Autodesk Fusion 360 part; units mm, degrees
(part 40 of 40)
  line L11757 (236.7591, 85.2532) -> (236.7374, 85.0889) construction
  line L11758 (236.7374, 85.0889) -> (236.7148, 84.9245) construction
  line L11759 (236.7148, 84.9245) -> (236.6913, 84.76) construction
  line L11760 (236.6913, 84.76) -> (236.667, 84.5954) construction
  line L11761 (236.667, 84.5954) -> (236.6418, 84.4308) construction
  line L11762 (236.6418, 84.4308) -> (236.6159, 84.266) construction
  line L11763 (236.6159, 84.266) -> (236.5891, 84.1013) construction
  line L11764 (236.5891, 84.1013) -> (236.5614, 83.9364) construction
  line L11765 (236.5614, 83.9364) -> (236.533, 83.7715) construction
  line L11766 (236.533, 83.7715) -> (236.5038, 83.6065) construction
  line L11767 (236.5038, 83.6065) -> (236.4737, 83.4415) construction
  line L11768 (236.4737, 83.4415) -> (236.4428, 83.2764) construction
  line L11769 (236.4428, 83.2764) -> (236.4112, 83.1113) construction
  line L11770 (236.4112, 83.1113) -> (236.3852, 82.9792) construction
  line L11771 (236.3852, 82.9792) -> (236.3654, 82.8801) construction
  line L11772 (236.3654, 82.8801) -> (236.352, 82.814) construction
  line L11773 (236.352, 82.814) -> (236.3452, 82.7809) construction
  arc A310 (232.0535, 81.3864) -> (236.3452, 82.7809) centre (212.132, 150) ccw
  arc A311 (170.3188, 110.6216) -> (172.7536, 108.1868) centre (212.132, 150) ccw
  arc A312 (144.9129, 174.2132) -> (143.5184, 169.9215) centre (212.132, 150) ccw
  arc A313 (253.9452, 189.3784) -> (251.5104, 191.8132) centre (212.132, 150) ccw
  arc A314 (204.8514, 206.9737) -> (201.4504, 206.435) centre (212.132, 150) ccw
  arc A315 (222.8136, 206.435) -> (219.4126, 206.9737) centre (212.132, 150) ccw
  arc A316 (269.1057, 157.2806) -> (268.567, 160.6816) centre (212.132, 150) ccw
  arc A317 (152.9878, 155.5428) -> (155.1583, 157.2806) centre (153.1745, 157.5341) ccw
  arc A318 (192.2105, 218.6136) -> (187.9188, 217.2191) centre (212.132, 150) ccw
  spline S157 degree 5 poles (272.9005, 155.6951) (272.9313, 155.6979) (272.9929, 155.7029) (273.0853, 155.7078) (273.2086, 155.7097) (273.363, 155.7056) (273.5176, 155.6969) (273.6723, 155.6854) (273.827, 155.6723) (273.9818, 155.6583) (274.1365, 155.6431) (274.2913, 155.6265) (274.446, 155.608) (274.6008, 155.5871) (274.7555, 155.5641) (274.9102, 155.539) (275.0649, 155.5121) (275.2195, 155.4838) (275.3741, 155.4542) (275.5286, 155.4233) (275.6831, 155.3913) (275.8375, 155.3579) (275.9918, 155.3232) (276.146, 155.2871) (276.3002, 155.2497) (276.4542, 155.2109) (276.6082, 155.1709) (276.7621, 155.1297) (276.9159, 155.0873) (277.0696, 155.0439) (277.2232, 154.9993) (277.3767, 154.9536) (277.53, 154.9068) (277.6833, 154.8589) (277.8364, 154.8099) (277.9894, 154.7599) (278.1423, 154.7087) (278.2951, 154.6566) (278.4478, 154.6035) (278.6003, 154.5493) (278.7526, 154.4942) (278.9049, 154.438) (279.057, 154.381) (279.209, 154.3229) (279.3608, 154.2639) (279.5124, 154.2039) (279.664, 154.143) (279.8153, 154.0812) (279.9665, 154.0185) (280.1176, 153.9548) (280.2685, 153.8903) (280.4192, 153.8249) (280.5698, 153.7585) (280.7202, 153.6913) (280.8704, 153.6233) (281.0205, 153.5543) (281.1704, 153.4846) (281.3201, 153.4139) (281.4696, 153.3425) (281.619, 153.2701) (281.7682, 153.197) (281.9172, 153.123) (282.066, 153.0482) (282.2146, 152.9726) (282.3631, 152.8962) (282.5113, 152.819) (282.6594, 152.741) (282.8072, 152.6622) (282.9549, 152.5826) (283.1023, 152.5023) (283.2496, 152.4211) (283.3672, 152.3556) (283.4554, 152.3061) (283.5141, 152.2729) (283.5435, 152.2563) knots 0 0 0 0 0 0 0.01428571 0.02857143 0.04285714 0.05714286 0.07142857 0.08571429 0.1 0.11428571 0.12857143 0.14285714 0.15714286 0.17142857 0.18571429 0.2 0.21428571 0.22857143 0.24285714 0.25714286 0.27142857 0.28571429 0.3 0.31428571 0.32857143 0.34285714 0.35714286 0.37142857 0.38571429 0.4 0.41428571 0.42857143 0.44285714 0.45714286 0.47142857 0.48571429 0.5 0.51428571 0.52857143 0.54285714 0.55714286 0.57142857 0.58571429 0.6 0.61428571 0.62857143 0.64285714 0.65714286 0.67142857 0.68571429 0.7 0.71428571 0.72857143 0.74285714 0.75714286 0.77142857 0.78571429 0.8 0.81428571 0.82857143 0.84285714 0.85714286 0.87142857 0.88571429 0.9 0.91428571 0.92857143 0.94285714 0.95714286 0.97142857 0.98571429 1 1 1 1 1 1
  line L11774 (272.9005, 155.6951) -> (272.9313, 155.6979) construction
  line L11775 (272.9313, 155.6979) -> (272.9929, 155.7029) construction
  line L11776 (272.9929, 155.7029) -> (273.0853, 155.7078) construction
  line L11777 (273.0853, 155.7078) -> (273.2086, 155.7097) construction
  line L11778 (273.2086, 155.7097) -> (273.363, 155.7056) construction
  line L11779 (273.363, 155.7056) -> (273.5176, 155.6969) construction
  line L11780 (273.5176, 155.6969) -> (273.6723, 155.6854) construction
  line L11781 (273.6723, 155.6854) -> (273.827, 155.6723) construction
  line L11782 (273.827, 155.6723) -> (273.9818, 155.6583) construction
  line L11783 (273.9818, 155.6583) -> (274.1365, 155.6431) construction
  line L11784 (274.1365, 155.6431) -> (274.2913, 155.6265) construction
  line L11785 (274.2913, 155.6265) -> (274.446, 155.608) construction
  line L11786 (274.446, 155.608) -> (274.6008, 155.5871) construction
  line L11787 (274.6008, 155.5871) -> (274.7555, 155.5641) construction
  line L11788 (274.7555, 155.5641) -> (274.9102, 155.539) construction
  line L11789 (274.9102, 155.539) -> (275.0649, 155.5121) construction
  line L11790 (275.0649, 155.5121) -> (275.2195, 155.4838) construction
  line L11791 (275.2195, 155.4838) -> (275.3741, 155.4542) construction
  line L11792 (275.3741, 155.4542) -> (275.5286, 155.4233) construction
  line L11793 (275.5286, 155.4233) -> (275.6831, 155.3913) construction
  line L11794 (275.6831, 155.3913) -> (275.8375, 155.3579) construction
  line L11795 (275.8375, 155.3579) -> (275.9918, 155.3232) construction
  line L11796 (275.9918, 155.3232) -> (276.146, 155.2871) construction
  line L11797 (276.146, 155.2871) -> (276.3002, 155.2497) construction
  line L11798 (276.3002, 155.2497) -> (276.4542, 155.2109) construction
  line L11799 (276.4542, 155.2109) -> (276.6082, 155.1709) construction
  line L11800 (276.6082, 155.1709) -> (276.7621, 155.1297) construction
  line L11801 (276.7621, 155.1297) -> (276.9159, 155.0873) construction
  line L11802 (276.9159, 155.0873) -> (277.0696, 155.0439) construction
  line L11803 (277.0696, 155.0439) -> (277.2232, 154.9993) construction
  line L11804 (277.2232, 154.9993) -> (277.3767, 154.9536) construction
  line L11805 (277.3767, 154.9536) -> (277.53, 154.9068) construction
  line L11806 (277.53, 154.9068) -> (277.6833, 154.8589) construction
  line L11807 (277.6833, 154.8589) -> (277.8364, 154.8099) construction
  line L11808 (277.8364, 154.8099) -> (277.9894, 154.7599) construction
  line L11809 (277.9894, 154.7599) -> (278.1423, 154.7087) construction
  line L11810 (278.1423, 154.7087) -> (278.2951, 154.6566) construction
  line L11811 (278.2951, 154.6566) -> (278.4478, 154.6035) construction
  line L11812 (278.4478, 154.6035) -> (278.6003, 154.5493) construction
  line L11813 (278.6003, 154.5493) -> (278.7526, 154.4942) construction
  line L11814 (278.7526, 154.4942) -> (278.9049, 154.438) construction
  line L11815 (278.9049, 154.438) -> (279.057, 154.381) construction
  line L11816 (279.057, 154.381) -> (279.209, 154.3229) construction
  line L11817 (279.209, 154.3229) -> (279.3608, 154.2639) construction
  line L11818 (279.3608, 154.2639) -> (279.5124, 154.2039) construction
  line L11819 (279.5124, 154.2039) -> (279.664, 154.143) construction
  line L11820 (279.664, 154.143) -> (279.8153, 154.0812) construction
  line L11821 (279.8153, 154.0812) -> (279.9665, 154.0185) construction
  line L11822 (279.9665, 154.0185) -> (280.1176, 153.9548) construction
  line L11823 (280.1176, 153.9548) -> (280.2685, 153.8903) construction
  line L11824 (280.2685, 153.8903) -> (280.4192, 153.8249) construction
  line L11825 (280.4192, 153.8249) -> (280.5698, 153.7585) construction
  line L11826 (280.5698, 153.7585) -> (280.7202, 153.6913) construction
  line L11827 (280.7202, 153.6913) -> (280.8704, 153.6233) construction
  line L11828 (280.8704, 153.6233) -> (281.0205, 153.5543) construction
  line L11829 (281.0205, 153.5543) -> (281.1704, 153.4846) construction
  line L11830 (281.1704, 153.4846) -> (281.3201, 153.4139) construction
  line L11831 (281.3201, 153.4139) -> (281.4696, 153.3425) construction
  line L11832 (281.4696, 153.3425) -> (281.619, 153.2701) construction
  line L11833 (281.619, 153.2701) -> (281.7682, 153.197) construction
  line L11834 (281.7682, 153.197) -> (281.9172, 153.123) construction
  line L11835 (281.9172, 153.123) -> (282.066, 153.0482) construction
  line L11836 (282.066, 153.0482) -> (282.2146, 152.9726) construction
  line L11837 (282.2146, 152.9726) -> (282.3631, 152.8962) construction
  line L11838 (282.3631, 152.8962) -> (282.5113, 152.819) construction
  line L11839 (282.5113, 152.819) -> (282.6594, 152.741) construction
  line L11840 (282.6594, 152.741) -> (282.8072, 152.6622) construction
  line L11841 (282.8072, 152.6622) -> (282.9549, 152.5826) construction
  line L11842 (282.9549, 152.5826) -> (283.1023, 152.5023) construction
  line L11843 (283.1023, 152.5023) -> (283.2496, 152.4211) construction
  line L11844 (283.2496, 152.4211) -> (283.3672, 152.3556) construction
  line L11845 (283.3672, 152.3556) -> (283.4554, 152.3061) construction
  line L11846 (283.4554, 152.3061) -> (283.5141, 152.2729) construction
  line L11847 (283.5141, 152.2729) -> (283.5435, 152.2563) construction
  arc A319 (172.7536, 191.8132) -> (170.3188, 189.3784) centre (212.132, 150) ccw
  arc A320 (160.1966, 125.4699) -> (161.7599, 122.4018) centre (212.132, 150) ccw
  arc A321 (155.697, 160.6816) -> (154.1697, 163.005) centre (153.7319, 161.0535) ccw
  spline S158 degree 5 poles (252.4583, 195.8153) (252.4787, 195.8385) (252.5188, 195.8854) (252.5771, 195.9573) (252.6512, 196.056) (252.7386, 196.1833) (252.8224, 196.3135) (252.904, 196.4454) (252.9844, 196.5782) (253.064, 196.7117) (253.1427, 196.8458) (253.2203, 196.9807) (253.2962, 197.1168) (253.3703, 197.2543) (253.4426, 197.393) (253.5133, 197.5329) (253.5824, 197.6738) (253.6504, 197.8156) (253.7173, 197.9581) (253.7832, 198.1012) (253.848, 198.245) (253.9118, 198.3895) (253.9744, 198.5347) (254.0359, 198.6807) (254.0962, 198.8274) (254.1554, 198.9749) (254.2135, 199.123) (254.2706, 199.2717) (254.3267, 199.421) (254.3819, 199.5709) (254.4361, 199.7214) (254.4894, 199.8724) (254.5417, 200.024) (254.593, 200.1761) (254.6434, 200.3288) (254.6928, 200.482) (254.7414, 200.6358) (254.789, 200.79) (254.8357, 200.9447) (254.8815, 201.0999) (254.9265, 201.2556) (254.9706, 201.4118) (255.0138, 201.5684) (255.0561, 201.7255) (255.0976, 201.883) (255.1383, 202.0409) (255.1781, 202.1993) (255.217, 202.3581) (255.2551, 202.5173) (255.2924, 202.6769) (255.3289, 202.8369) (255.3646, 202.9973) (255.3994, 203.1581) (255.4335, 203.3193) (255.4667, 203.4809) (255.4992, 203.6428) (255.5308, 203.8051) (255.5617, 203.9677) (255.5917, 204.1307) (255.621, 204.294) (255.6495, 204.4577) (255.6773, 204.6217) (255.7043, 204.7861) (255.7304, 204.9508) (255.7559, 205.1158) (255.7806, 205.2811) (255.8045, 205.4467) (255.8276, 205.6126) (255.85, 205.7789) (255.8717, 205.9454) (255.8926, 206.1122) (255.9087, 206.2459) (255.9205, 206.3463) (255.9282, 206.4133) (255.932, 206.4469) knots 0 0 0 0 0 0 0.01428571 0.02857143 0.04285714 0.05714286 0.07142857 0.08571429 0.1 0.11428571 0.12857143 0.14285714 0.15714286 0.17142857 0.18571429 0.2 0.21428571 0.22857143 0.24285714 0.25714286 0.27142857 0.28571429 0.3 0.31428571 0.32857143 0.34285714 0.35714286 0.37142857 0.38571429 0.4 0.41428571 0.42857143 0.44285714 0.45714286 0.47142857 0.48571429 0.5 0.51428571 0.52857143 0.54285714 0.55714286 0.57142857 0.58571429 0.6 0.61428571 0.62857143 0.64285714 0.65714286 0.67142857 0.68571429 0.7 0.71428571 0.72857143 0.74285714 0.75714286 0.77142857 0.78571429 0.8 0.81428571 0.82857143 0.84285714 0.85714286 0.87142857 0.88571429 0.9 0.91428571 0.92857143 0.94285714 0.95714286 0.97142857 0.98571429 1 1 1 1 1 1
  line L11848 (252.4583, 195.8153) -> (252.4787, 195.8385) construction
  line L11849 (252.4787, 195.8385) -> (252.5188, 195.8854) construction
  line L11850 (252.5188, 195.8854) -> (252.5771, 195.9573) construction
  line L11851 (252.5771, 195.9573) -> (252.6512, 196.056) construction
  line L11852 (252.6512, 196.056) -> (252.7386, 196.1833) construction
  line L11853 (252.7386, 196.1833) -> (252.8224, 196.3135) construction
  line L11854 (252.8224, 196.3135) -> (252.904, 196.4454) construction
  line L11855 (252.904, 196.4454) -> (252.9844, 196.5782) construction
  line L11856 (252.9844, 196.5782) -> (253.064, 196.7117) construction
  line L11857 (253.064, 196.7117) -> (253.1427, 196.8458) construction
  line L11858 (253.1427, 196.8458) -> (253.2203, 196.9807) construction
  line L11859 (253.2203, 196.9807) -> (253.2962, 197.1168) construction
  line L11860 (253.2962, 197.1168) -> (253.3703, 197.2543) construction
  line L11861 (253.3703, 197.2543) -> (253.4426, 197.393) construction
  line L11862 (253.4426, 197.393) -> (253.5133, 197.5329) construction
  line L11863 (253.5133, 197.5329) -> (253.5824, 197.6738) construction
  line L11864 (253.5824, 197.6738) -> (253.6504, 197.8156) construction
  line L11865 (253.6504, 197.8156) -> (253.7173, 197.9581) construction
  line L11866 (253.7173, 197.9581) -> (253.7832, 198.1012) construction
  line L11867 (253.7832, 198.1012) -> (253.848, 198.245) construction
  line L11868 (253.848, 198.245) -> (253.9118, 198.3895) construction
  line L11869 (253.9118, 198.3895) -> (253.9744, 198.5347) construction
  line L11870 (253.9744, 198.5347) -> (254.0359, 198.6807) construction
  line L11871 (254.0359, 198.6807) -> (254.0962, 198.8274) construction
  line L11872 (254.0962, 198.8274) -> (254.1554, 198.9749) construction
  line L11873 (254.1554, 198.9749) -> (254.2135, 199.123) construction
  line L11874 (254.2135, 199.123) -> (254.2706, 199.2717) construction
  line L11875 (254.2706, 199.2717) -> (254.3267, 199.421) construction
  line L11876 (254.3267, 199.421) -> (254.3819, 199.5709) construction
  line L11877 (254.3819, 199.5709) -> (254.4361, 199.7214) construction
  line L11878 (254.4361, 199.7214) -> (254.4894, 199.8724) construction
  line L11879 (254.4894, 199.8724) -> (254.5417, 200.024) construction
  line L11880 (254.5417, 200.024) -> (254.593, 200.1761) construction
  line L11881 (254.593, 200.1761) -> (254.6434, 200.3288) construction
  line L11882 (254.6434, 200.3288) -> (254.6928, 200.482) construction
  line L11883 (254.6928, 200.482) -> (254.7414, 200.6358) construction
  line L11884 (254.7414, 200.6358) -> (254.789, 200.79) construction
  line L11885 (254.789, 200.79) -> (254.8357, 200.9447) construction
  line L11886 (254.8357, 200.9447) -> (254.8815, 201.0999) construction
  line L11887 (254.8815, 201.0999) -> (254.9265, 201.2556) construction
  line L11888 (254.9265, 201.2556) -> (254.9706, 201.4118) construction
  line L11889 (254.9706, 201.4118) -> (255.0138, 201.5684) construction
  line L11890 (255.0138, 201.5684) -> (255.0561, 201.7255) construction
  line L11891 (255.0561, 201.7255) -> (255.0976, 201.883) construction
  line L11892 (255.0976, 201.883) -> (255.1383, 202.0409) construction
  line L11893 (255.1383, 202.0409) -> (255.1781, 202.1993) construction
  line L11894 (255.1781, 202.1993) -> (255.217, 202.3581) construction
  line L11895 (255.217, 202.3581) -> (255.2551, 202.5173) construction
  line L11896 (255.2551, 202.5173) -> (255.2924, 202.6769) construction
  line L11897 (255.2924, 202.6769) -> (255.3289, 202.8369) construction
  line L11898 (255.3289, 202.8369) -> (255.3646, 202.9973) construction
  line L11899 (255.3646, 202.9973) -> (255.3994, 203.1581) construction
  line L11900 (255.3994, 203.1581) -> (255.4335, 203.3193) construction
  line L11901 (255.4335, 203.3193) -> (255.4667, 203.4809) construction
  line L11902 (255.4667, 203.4809) -> (255.4992, 203.6428) construction
  line L11903 (255.4992, 203.6428) -> (255.5308, 203.8051) construction
  line L11904 (255.5308, 203.8051) -> (255.5617, 203.9677) construction
  line L11905 (255.5617, 203.9677) -> (255.5917, 204.1307) construction
  line L11906 (255.5917, 204.1307) -> (255.621, 204.294) construction
  line L11907 (255.621, 204.294) -> (255.6495, 204.4577) construction
  line L11908 (255.6495, 204.4577) -> (255.6773, 204.6217) construction
  line L11909 (255.6773, 204.6217) -> (255.7043, 204.7861) construction
  line L11910 (255.7043, 204.7861) -> (255.7304, 204.9508) construction
  line L11911 (255.7304, 204.9508) -> (255.7559, 205.1158) construction
  line L11912 (255.7559, 205.1158) -> (255.7806, 205.2811) construction
  line L11913 (255.7806, 205.2811) -> (255.8045, 205.4467) construction
  line L11914 (255.8045, 205.4467) -> (255.8276, 205.6126) construction
  line L11915 (255.8276, 205.6126) -> (255.85, 205.7789) construction
  line L11916 (255.85, 205.7789) -> (255.8717, 205.9454) construction
  line L11917 (255.8717, 205.9454) -> (255.8926, 206.1122) construction
  line L11918 (255.8926, 206.1122) -> (255.9087, 206.2459) construction
  line L11919 (255.9087, 206.2459) -> (255.9205, 206.3463) construction
  line L11920 (255.9205, 206.3463) -> (255.9282, 206.4133) construction
  line L11921 (255.9282, 206.4133) -> (255.932, 206.4469) construction
  arc A322 (268.567, 139.3184) -> (270.0943, 136.995) centre (270.5321, 138.9465) ccw
  line L11922 (206.5892, 209.1442) -> (206.4369, 210.7685)
  line L11923 (235.6801, 204.5366) -> (236.3268, 206.0345)
  line L11924 (270.0943, 136.995) -> (271.6862, 136.6378)
  line L11925 (266.6686, 126.4519) -> (268.1665, 125.8052)
  arc A323 (170.3188, 110.6216) -> (172.7536, 108.1868) centre (212.132, 150) ccw
  spline S159 degree 5 poles (217.8271, 210.7685) (217.8299, 210.7993) (217.8349, 210.8609) (217.8398, 210.9533) (217.8417, 211.0766) (217.8376, 211.231) (217.8289, 211.3856) (217.8174, 211.5403) (217.8043, 211.695) (217.7903, 211.8498) (217.7751, 212.0045) (217.7585, 212.1593) (217.74, 212.314) (217.7191, 212.4688) (217.6961, 212.6235) (217.671, 212.7782) (217.6441, 212.9329) (217.6158, 213.0875) (217.5862, 213.2421) (217.5553, 213.3966) (217.5233, 213.5511) (217.4899, 213.7055) (217.4552, 213.8598) (217.4191, 214.014) (217.3817, 214.1682) (217.3429, 214.3222) (217.3029, 214.4762) (217.2617, 214.6301) (217.2193, 214.7839) (217.1759, 214.9376) (217.1313, 215.0912) (217.0856, 215.2447) (217.0388, 215.398) (216.9909, 215.5513) (216.9419, 215.7044) (216.8919, 215.8574) (216.8407, 216.0103) (216.7886, 216.1631) (216.7355, 216.3158) (216.6813, 216.4683) (216.6262, 216.6206) (216.57, 216.7729) (216.513, 216.925) (216.4549, 217.077) (216.3959, 217.2288) (216.3359, 217.3804) (216.275, 217.532) (216.2132, 217.6833) (216.1505, 217.8345) (216.0868, 217.9856) (216.0223, 218.1365) (215.9569, 218.2872) (215.8905, 218.4378) (215.8233, 218.5882) (215.7553, 218.7384) (215.6863, 218.8885) (215.6166, 219.0384) (215.5459, 219.1881) (215.4745, 219.3376) (215.4021, 219.487) (215.329, 219.6362) (215.255, 219.7852) (215.1802, 219.934) (215.1046, 220.0826) (215.0282, 220.2311) (214.951, 220.3793) (214.873, 220.5274) (214.7942, 220.6752) (214.7146, 220.8229) (214.6343, 220.9703) (214.5531, 221.1176) (214.4876, 221.2352) (214.4381, 221.3234) (214.4049, 221.3821) (214.3883, 221.4115) knots 0 0 0 0 0 0 0.01428571 0.02857143 0.04285714 0.05714286 0.07142857 0.08571429 0.1 0.11428571 0.12857143 0.14285714 0.15714286 0.17142857 0.18571429 0.2 0.21428571 0.22857143 0.24285714 0.25714286 0.27142857 0.28571429 0.3 0.31428571 0.32857143 0.34285714 0.35714286 0.37142857 0.38571429 0.4 0.41428571 0.42857143 0.44285714 0.45714286 0.47142857 0.48571429 0.5 0.51428571 0.52857143 0.54285714 0.55714286 0.57142857 0.58571429 0.6 0.61428571 0.62857143 0.64285714 0.65714286 0.67142857 0.68571429 0.7 0.71428571 0.72857143 0.74285714 0.75714286 0.77142857 0.78571429 0.8 0.81428571 0.82857143 0.84285714 0.85714286 0.87142857 0.88571429 0.9 0.91428571 0.92857143 0.94285714 0.95714286 0.97142857 0.98571429 1 1 1 1 1 1
  line L11926 (217.8271, 210.7685) -> (217.8299, 210.7993) construction
  line L11927 (217.8299, 210.7993) -> (217.8349, 210.8609) construction
  line L11928 (217.8349, 210.8609) -> (217.8398, 210.9533) construction
  line L11929 (217.8398, 210.9533) -> (217.8417, 211.0766) construction
  line L11930 (217.8417, 211.0766) -> (217.8376, 211.231) construction
  line L11931 (217.8376, 211.231) -> (217.8289, 211.3856) construction
  line L11932 (217.8289, 211.3856) -> (217.8174, 211.5403) construction
  line L11933 (217.8174, 211.5403) -> (217.8043, 211.695) construction
  line L11934 (217.8043, 211.695) -> (217.7903, 211.8498) construction
  line L11935 (217.7903, 211.8498) -> (217.7751, 212.0045) construction
  line L11936 (217.7751, 212.0045) -> (217.7585, 212.1593) construction
  line L11937 (217.7585, 212.1593) -> (217.74, 212.314) construction
  line L11938 (217.74, 212.314) -> (217.7191, 212.4688) construction
  line L11939 (217.7191, 212.4688) -> (217.6961, 212.6235) construction
  line L11940 (217.6961, 212.6235) -> (217.671, 212.7782) construction
  line L11941 (217.671, 212.7782) -> (217.6441, 212.9329) construction
  line L11942 (217.6441, 212.9329) -> (217.6158, 213.0875) construction
  line L11943 (217.6158, 213.0875) -> (217.5862, 213.2421) construction
  line L11944 (217.5862, 213.2421) -> (217.5553, 213.3966) construction
  line L11945 (217.5553, 213.3966) -> (217.5233, 213.5511) construction
  line L11946 (217.5233, 213.5511) -> (217.4899, 213.7055) construction
  line L11947 (217.4899, 213.7055) -> (217.4552, 213.8598) construction
  line L11948 (217.4552, 213.8598) -> (217.4191, 214.014) construction
  line L11949 (217.4191, 214.014) -> (217.3817, 214.1682) construction
  line L11950 (217.3817, 214.1682) -> (217.3429, 214.3222) construction
  line L11951 (217.3429, 214.3222) -> (217.3029, 214.4762) construction
  line L11952 (217.3029, 214.4762) -> (217.2617, 214.6301) construction
  line L11953 (217.2617, 214.6301) -> (217.2193, 214.7839) construction
  line L11954 (217.2193, 214.7839) -> (217.1759, 214.9376) construction
  line L11955 (217.1759, 214.9376) -> (217.1313, 215.0912) construction
  line L11956 (217.1313, 215.0912) -> (217.0856, 215.2447) construction
  line L11957 (217.0856, 215.2447) -> (217.0388, 215.398) construction
  line L11958 (217.0388, 215.398) -> (216.9909, 215.5513) construction
  line L11959 (216.9909, 215.5513) -> (216.9419, 215.7044) construction
  line L11960 (216.9419, 215.7044) -> (216.8919, 215.8574) construction
  line L11961 (216.8919, 215.8574) -> (216.8407, 216.0103) construction
  line L11962 (216.8407, 216.0103) -> (216.7886, 216.1631) construction
  line L11963 (216.7886, 216.1631) -> (216.7355, 216.3158) construction
  line L11964 (216.7355, 216.3158) -> (216.6813, 216.4683) construction
  line L11965 (216.6813, 216.4683) -> (216.6262, 216.6206) construction
  line L11966 (216.6262, 216.6206) -> (216.57, 216.7729) construction
  line L11967 (216.57, 216.7729) -> (216.513, 216.925) construction
  line L11968 (216.513, 216.925) -> (216.4549, 217.077) construction
  line L11969 (216.4549, 217.077) -> (216.3959, 217.2288) construction
  line L11970 (216.3959, 217.2288) -> (216.3359, 217.3804) construction
  line L11971 (216.3359, 217.3804) -> (216.275, 217.532) construction
  line L11972 (216.275, 217.532) -> (216.2132, 217.6833) construction
  line L11973 (216.2132, 217.6833) -> (216.1505, 217.8345) construction
  line L11974 (216.1505, 217.8345) -> (216.0868, 217.9856) construction
  line L11975 (216.0868, 217.9856) -> (216.0223, 218.1365) construction
  line L11976 (216.0223, 218.1365) -> (215.9569, 218.2872) construction
  line L11977 (215.9569, 218.2872) -> (215.8905, 218.4378) construction
  line L11978 (215.8905, 218.4378) -> (215.8233, 218.5882) construction
  line L11979 (215.8233, 218.5882) -> (215.7553, 218.7384) construction
  line L11980 (215.7553, 218.7384) -> (215.6863, 218.8885) construction
  line L11981 (215.6863, 218.8885) -> (215.6166, 219.0384) construction
  line L11982 (215.6166, 219.0384) -> (215.5459, 219.1881) construction
  line L11983 (215.5459, 219.1881) -> (215.4745, 219.3376) construction
  line L11984 (215.4745, 219.3376) -> (215.4021, 219.487) construction
  line L11985 (215.4021, 219.487) -> (215.329, 219.6362) construction
  line L11986 (215.329, 219.6362) -> (215.255, 219.7852) construction
  line L11987 (215.255, 219.7852) -> (215.1802, 219.934) construction
  line L11988 (215.1802, 219.934) -> (215.1046, 220.0826) construction
  line L11989 (215.1046, 220.0826) -> (215.0282, 220.2311) construction
  line L11990 (215.0282, 220.2311) -> (214.951, 220.3793) construction
  line L11991 (214.951, 220.3793) -> (214.873, 220.5274) construction
  line L11992 (214.873, 220.5274) -> (214.7942, 220.6752) construction
  line L11993 (214.7942, 220.6752) -> (214.7146, 220.8229) construction
  line L11994 (214.7146, 220.8229) -> (214.6343, 220.9703) construction
  line L11995 (214.6343, 220.9703) -> (214.5531, 221.1176) construction
  line L11996 (214.5531, 221.1176) -> (214.4876, 221.2352) construction
  line L11997 (214.4876, 221.2352) -> (214.4381, 221.3234) construction
  line L11998 (214.4381, 221.3234) -> (214.4049, 221.3821) construction
  line L11999 (214.4049, 221.3821) -> (214.3883, 221.4115) construction
sketch "Base Circle (2)" plane through (0, 0, 0) normal (0, 0, 1) x (1, 0, 0)
  circle A0 centre (0, 0) radius 57.437
  circle A1 centre (0, 0) radius 2.3
extrude "Extrude2" [suppressed]
sketch "Gear Tooth (2)" plane through (0, 0, 0) normal (0, 0, 1) x (1, 0, 0)
  spline S0 degree 5 poles (60.7685, -5.6951) (60.7993, -5.6979) (60.8609, -5.7029) (60.9533, -5.7078) (61.0766, -5.7097) (61.231, -5.7056) (61.3856, -5.6969) (61.5403, -5.6854) (61.695, -5.6723) (61.8498, -5.6583) (62.0045, -5.6431) (62.1593, -5.6265) (62.314, -5.608) (62.4688, -5.5871) (62.6235, -5.5641) (62.7782, -5.539) (62.9329, -5.5121) (63.0875, -5.4838) (63.2421, -5.4542) (63.3966, -5.4233) (63.5511, -5.3913) (63.7055, -5.3579) (63.8598, -5.3232) (64.014, -5.2871) (64.1682, -5.2497) (64.3222, -5.2109) (64.4762, -5.1709) (64.6301, -5.1297) (64.7839, -5.0873) (64.9376, -5.0439) (65.0912, -4.9993) (65.2447, -4.9536) (65.398, -4.9068) (65.5513, -4.8589) (65.7044, -4.8099) (65.8574, -4.7599) (66.0103, -4.7087) (66.1631, -4.6566) (66.3158, -4.6035) (66.4683, -4.5493) (66.6206, -4.4942) (66.7729, -4.438) (66.925, -4.381) (67.077, -4.3229) (67.2288, -4.2639) (67.3804, -4.2039) (67.532, -4.143) (67.6833, -4.0812) (67.8345, -4.0185) (67.9856, -3.9548) (68.1365, -3.8903) (68.2872, -3.8249) (68.4378, -3.7585) (68.5882, -3.6913) (68.7384, -3.6233) (68.8885, -3.5543) (69.0384, -3.4846) (69.1881, -3.4139) (69.3376, -3.3425) (69.487, -3.2701) (69.6362, -3.197) (69.7852, -3.123) (69.934, -3.0482) (70.0826, -2.9726) (70.2311, -2.8962) (70.3793, -2.819) (70.5274, -2.741) (70.6752, -2.6622) (70.8229, -2.5826) (70.9703, -2.5023) (71.1176, -2.4211) (71.2352, -2.3556) (71.3234, -2.3061) (71.3821, -2.2729) (71.4115, -2.2563) knots 0 0 0 0 0 0 0.01428571 0.02857143 0.04285714 0.05714286 0.07142857 0.08571429 0.1 0.11428571 0.12857143 0.14285714 0.15714286 0.17142857 0.18571429 0.2 0.21428571 0.22857143 0.24285714 0.25714286 0.27142857 0.28571429 0.3 0.31428571 0.32857143 0.34285714 0.35714286 0.37142857 0.38571429 0.4 0.41428571 0.42857143 0.44285714 0.45714286 0.47142857 0.48571429 0.5 0.51428571 0.52857143 0.54285714 0.55714286 0.57142857 0.58571429 0.6 0.61428571 0.62857143 0.64285714 0.65714286 0.67142857 0.68571429 0.7 0.71428571 0.72857143 0.74285714 0.75714286 0.77142857 0.78571429 0.8 0.81428571 0.82857143 0.84285714 0.85714286 0.87142857 0.88571429 0.9 0.91428571 0.92857143 0.94285714 0.95714286 0.97142857 0.98571429 1 1 1 1 1 1
  spline S1 degree 5 poles (60.7685, 5.6951) (60.7993, 5.6979) (60.8609, 5.7029) (60.9533, 5.7078) (61.0766, 5.7097) (61.231, 5.7056) (61.3856, 5.6969) (61.5403, 5.6854) (61.695, 5.6723) (61.8498, 5.6583) (62.0045, 5.6431) (62.1593, 5.6265) (62.314, 5.608) (62.4688, 5.5871) (62.6235, 5.5641) (62.7782, 5.539) (62.9329, 5.5121) (63.0875, 5.4838) (63.2421, 5.4542) (63.3966, 5.4233) (63.5511, 5.3913) (63.7055, 5.3579) (63.8598, 5.3232) (64.014, 5.2871) (64.1682, 5.2497) (64.3222, 5.2109) (64.4762, 5.1709) (64.6301, 5.1297) (64.7839, 5.0873) (64.9376, 5.0439) (65.0912, 4.9993) (65.2447, 4.9536) (65.398, 4.9068) (65.5513, 4.8589) (65.7044, 4.8099) (65.8574, 4.7599) (66.0103, 4.7087) (66.1631, 4.6566) (66.3158, 4.6035) (66.4683, 4.5493) (66.6206, 4.4942) (66.7729, 4.438) (66.925, 4.381) (67.077, 4.3229) (67.2288, 4.2639) (67.3804, 4.2039) (67.532, 4.143) (67.6833, 4.0812) (67.8345, 4.0185) (67.9856, 3.9548) (68.1365, 3.8903) (68.2872, 3.8249) (68.4378, 3.7585) (68.5882, 3.6913) (68.7384, 3.6233) (68.8885, 3.5543) (69.0384, 3.4846) (69.1881, 3.4139) (69.3376, 3.3425) (69.487, 3.2701) (69.6362, 3.197) (69.7852, 3.123) (69.934, 3.0482) (70.0826, 2.9726) (70.2311, 2.8962) (70.3793, 2.819) (70.5274, 2.741) (70.6752, 2.6622) (70.8229, 2.5826) (70.9703, 2.5023) (71.1176, 2.4211) (71.2352, 2.3556) (71.3234, 2.3061) (71.3821, 2.2729) (71.4115, 2.2563) knots 0 0 0 0 0 0 0.01428571 0.02857143 0.04285714 0.05714286 0.07142857 0.08571429 0.1 0.11428571 0.12857143 0.14285714 0.15714286 0.17142857 0.18571429 0.2 0.21428571 0.22857143 0.24285714 0.25714286 0.27142857 0.28571429 0.3 0.31428571 0.32857143 0.34285714 0.35714286 0.37142857 0.38571429 0.4 0.41428571 0.42857143 0.44285714 0.45714286 0.47142857 0.48571429 0.5 0.51428571 0.52857143 0.54285714 0.55714286 0.57142857 0.58571429 0.6 0.61428571 0.62857143 0.64285714 0.65714286 0.67142857 0.68571429 0.7 0.71428571 0.72857143 0.74285714 0.75714286 0.77142857 0.78571429 0.8 0.81428571 0.82857143 0.84285714 0.85714286 0.87142857 0.88571429 0.9 0.91428571 0.92857143 0.94285714 0.95714286 0.97142857 0.98571429 1 1 1 1 1 1
  arc A0 (71.4115, -2.2563) -> (71.4115, 2.2563) centre (0, 0) ccw
  line L0 (57.1764, -5.3584) -> (60.7685, -5.6951)
  line L1 (57.1764, 5.3584) -> (60.7685, 5.6951)
  line L2 (57.1764, -5.3584) -> (57.1764, 5.3584)
  point P0 (61.5163, -5.6869)
  point P1 (62.2698, -5.6129)
  point P2 (63.027, -5.4947)
  point P3 (63.7867, -5.3395)
  point P4 (64.5483, -5.1514)
  point P5 (65.3112, -4.9332)
  point P6 (66.075, -4.6865)
  point P7 (66.8392, -4.413)
  point P8 (67.6034, -4.1137)
  point P9 (68.3672, -3.7895)
  point P10 (69.1303, -3.4411)
  point P11 (69.8923, -3.0691)
  point P12 (70.6528, -2.674)
  point P13 (61.5163, 5.6869)
  point P14 (62.2698, 5.6129)
  point P15 (63.027, 5.4947)
  point P16 (63.7867, 5.3395)
  point P17 (64.5483, 5.1514)
  point P18 (65.3112, 4.9332)
  point P19 (66.075, 4.6865)
  point P20 (66.8392, 4.413)
  point P21 (67.6034, 4.1137)
  point P22 (68.3672, 3.7895)
  point P23 (69.1303, 3.4411)
  point P24 (69.8923, 3.0691)
  point P25 (70.6528, 2.674)
extrude "Extrude3" [suppressed]
fillet "Fillet1" [suppressed]
pattern_circular "C-Pattern1" [suppressed]
sketch "Diametrial Pitch Circle (2)" plane through (0, 0, 0) normal (0, 0, 1) x (1, 0, 0)
  circle A0 centre (0, 0) radius 64.9519 construction
hidden bodies 1 2 3 4 5 6
equation "d1 = 2 * ( small_arm + edge_buffer )"
equation "small_arm = 50 mm"
equation "edge_buffer = 10 mm"
equation "d4 = 2 * small_arm"
equation "stick_diameter = 4.6 mm"
equation "d6 = stick_diameter"
equation "d7 = stick_diameter"
equation "d8 = small_arm * 2"
equation "arm_buffer = 5 mm"
equation "arm_width = 10 mm"
equation "d11 = small_arm + ( 2 * arm_buffer )"
equation "d12 = arm_width"
equation "d13 = small_arm / 2"
equation "d14 = small_arm / 2"
equation "d15 = stick_diameter"
equation "d16 = stick_diameter"
equation "thick_1 = 4.2 mm"
equation "d18 = small_arm + ( small_arm * 2 )"
equation "long_arm = small_arm * 3"
equation "d20 = long_arm + ( 2 * arm_buffer )"
equation "d21 = arm_width"
equation "d22 = long_arm / 2"
equation "d23 = long_arm / 2"
equation "d24 = stick_diameter"
equation "d25 = stick_diameter"
equation "d26 = small_arm"
equation "d27 = arm_width * 2"
equation "d28 = arm_width"
equation "d29 = long_arm"
equation "d30 = long_arm * 1.5"
equation "d31 = arm_width"
equation "d32 = long_arm * 1.5"
equation "d33 = arm_width"
equation "d34 = stick_diameter"
equation "d35 = thick_1"
equation "center_spacing = 10 mm"
equation "teeth = 20"
equation "module_num = sqrt(42.1875)"
equation "epsilon = 12.132 mm"
equation "d41 = ( 4 * small_arm ) + epsilon"
equation "d42 = 3 * small_arm"
equation "d43 = sqrt(( 4 * small_arm + epsilon ) ^ 2 + ( 3 * small_arm ) ^ 2)"
equation "d44 = small_arm"
equation "d45 = small_arm * 2"
equation "d46 = small_arm * 6"
equation "d47 = small_arm * 6"
equation "d48 = stick_diameter"
equation "d49 = stick_diameter"
equation "d50 = stick_diameter"
equation "d60 = small_arm"
equation "d74 = stick_diameter"
equation "d75 = stick_diameter"
equation "d76 = arm_width"
equation "d82 = arm_width * 2"
equation "d83 = arm_width"
equation "d84 = stick_diameter"
equation "d85 = stick_diameter"
equation "d87 = small_arm * 1.5"
equation "d88 = arm_width"
named bodies: "Spur Gear (20 teeth)"
